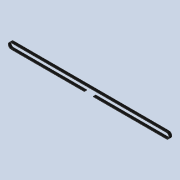
# Autodesk Inventor part: 0005-10-1015 curea x
Saved by Autodesk Inventor 2020 (Build 240168000, 168)
## iProperties
Created: 2020-12-19
Part Number: 0005-10-1015 curea x
Material: Generic
Document SubType Name: Modeling
Designer: Iulian Bors
Density: 1 g/cm^3
Appearance: Default(1)
Author: Iulian Bors
Subject: 10-1015
Autodesk Inventor part; units mm, degrees
ref_plane "YZ Plane" through (0, 0, 0) normal (1, 0, 0) x (0, 1, 0)
ref_plane "XZ Plane" through (0, 0, 0) normal (0, 1, 0) x (-1, 0, 0)
ref_plane "XY Plane" through (0, 0, 0) normal (0, 0, 1) x (1, 0, 0)
sketch "Sketch1" plane through (0, 0, 0) normal (0, 0, 1) x (1, 0, 0)
  line L0 (-260.6545, 0) -> (94.3455, 0) construction
  line L1 (-260.6545, -6) -> (94.3455, -6)
  line L2 (94.3455, 6) -> (-260.6545, 6)
  arc A0 (-260.6545, 6) -> (-260.6545, -6) centre (-260.6545, 0) ccw
  arc A1 (94.3455, -6) -> (94.3455, 6) centre (94.3455, 0) ccw
  line L3 (-260.6545, 7) -> (94.3455, 7)
  arc A2 (94.3455, -7) -> (94.3455, 7) centre (94.3455, 0) ccw
  line L4 (94.3455, -7) -> (-260.6545, -7)
  arc A3 (-260.6545, 7) -> (-260.6545, -7) centre (-260.6545, 0) ccw
  point P0 (0, 0)
  point P1 (-83.1545, 0)
  dimension "d0" = 355
  dimension "d1" = 12
  dimension "d2" = 1
  constraints: 12 end point, 8 point on circle, 4 centre point, 4 tangent, 2 parallel, 1 horizontal, 1 midpoint, 3 other
  measures "d0" distance of L0.start L0.end
  measures "d1" distance between parallel lines of L1 L2
  measures "d2" distance between parallel lines of L2 L3
extrude "Extrusion1" add sketch "Sketch1" along normal mid plane 6
sketch "Sketch2" plane through (-260.6545, -7, -3) normal (0, -1, 0) x (1, 0, 0)
  line L0 (206.0244, 13.746) -> (201.5244, 13.746) projected
  line L1 (0, 6) -> (355, 6) projected
  line L2 (355, 0) -> (0, 0) projected
  line L3 (167.5, 6) -> (187.5, 6)
  line L4 (187.5, 6) -> (187.5, 0)
  line L5 (187.5, 0) -> (167.5, 0)
  line L6 (167.5, 0) -> (167.5, 6)
  point P0 (177.5, 6)
  point P1 (177.5, 6)
  point P2 (167.5, 6)
  point P3 (167.5, 0)
  point P4 (187.5, 0)
  dimension "d11" = 20
  constraints: 8 end point, 2 collinear, 2 midpoint, 2 parallel, 1 coincident, 1 horizontal, 1 perpendicular
  measures "d11" distance of L3.start L3.end
extrude "Extrusion2" cut sketch "Sketch2" against normal blind 6.75
sketch "Sketch8" plane through (-93.1545, -7, 3) normal (1, 0, 0) x (0, 0, -1)
  line L0 (0, 1) -> (6, 1) projected
  line L1 (0, 0) -> (0, 1) projected
  line L2 (6, 0) -> (0, 0) projected
  line L3 (6, 1) -> (6, 0) projected
  point P0 (3, 7)
sketch "Sketch7" plane through (0, 0, 0) normal (0, 0, 1) x (1, 0, 0)
  line L0 (-93.1545, -6) -> (-93.1545, -7) projected
  line L1 (-93.1545, -6.5) -> (-89.8271, -9.4837) construction
  line L2 (-89.8271, -9.4837) -> (-86.2682, -8.1641) construction
  line L3 (-86.2682, -8.1641) -> (-79.2288, -4.4453) construction
  line L4 (-79.2288, -4.4453) -> (-81.5081, -1.2462) construction
  line L5 (-81.5081, -1.2462) -> (-85.9068, -0.2066) construction
  line L6 (-85.9068, -0.2066) -> (-88.9858, -2.4459) construction
  line L7 (-88.9858, -2.4459) -> (-90.3854, -5.165) construction
  line L8 (-260.6545, -6) -> (-93.1545, -6) projected
  line L9 (-90.3854, -5.165) -> (-92.5447, -6) construction
  spline S0 degree 4 poles (-93.1545, -6.5) (-89.8271, -9.4837) (-86.2682, -8.1641) (-79.2288, -4.4453) (-81.5081, -1.2462) (-85.9068, -0.2066) (-88.9858, -2.4459) (-90.3854, -5.165) (-92.5447, -6) knots 1 1 1 1 1 2 3 4 5 6 6 6 6 6
  point P0 (0, 0)
  constraints: 1 midpoint, 1 point on line, 3 other
sweep "Sweep3" add profiles "Sketch8" path "Sketch7" separate body path curves S0
sketch "Sketch9" plane through (0, 0, 0) normal (0, 0, 1) x (1, 0, 0)
  line L0 (-73.1545, -6) -> (-73.1545, -7) projected
  line L1 (-73.1545, -6.5) -> (-76.1323, -6.5) construction
  line L2 (-76.1323, -6.5) -> (-78.6484, -3.6505) construction
  line L3 (-78.6484, -3.6505) -> (-78.6484, 0) construction
  line L4 (-78.6484, 0) -> (-75.0222, 2.0479) construction
  line L5 (-75.0222, 2.0479) -> (-70.9519, 3.306) construction
  line L6 (-70.9519, 3.306) -> (-67.6217, -1.5783) construction
  line L7 (-67.6217, -1.5783) -> (-63.9955, -5.4266) construction
  line L8 (-63.9955, -5.4266) -> (-58.5191, -4.9825) construction
  spline S0 degree 4 poles (-73.1545, -6.5) (-76.1323, -6.5) (-78.6484, -3.6505) (-78.6484, 0) (-75.0222, 2.0479) (-70.9519, 3.306) (-67.6217, -1.5783) (-63.9955, -5.4266) (-58.5191, -4.9825) knots 1 1 1 1 1 2 3 4 5 6 6 6 6 6
  point P0 (0, 0)
  constraints: 1 midpoint, 1 perpendicular, 1 vertical, 3 other
sketch "Sketch10" plane through (-73.1545, -7, -3) normal (-1, 0, 0) x (0, 0, 1)
  line L0 (0, 1) -> (6, 1) projected
  line L1 (0, 0) -> (0, 1) projected
  line L2 (6, 0) -> (0, 0) projected
  line L3 (6, 1) -> (6, 0) projected
  point P0 (3, 7)
sweep "Sweep4" add profiles "Sketch10" path "Sketch9" separate body path curves S0
body "Solid1"
body "Solid4"
body "Solid5"
